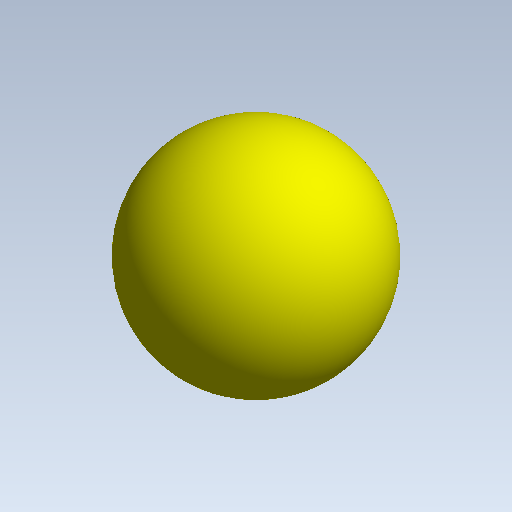
# Autodesk Inventor part: 17-40-27.4-12-ybrg1-43-6.747-28.5
Saved by Autodesk Inventor 2020 (Build 240168000, 168)
## iProperties
Part Number: 17-40-27.4-12-ybrg1-43-6.747-28.5
Material: Generic
Catalog Web Link: www.cadenas.de
Description: Ball for Y units-Y-bearings
Vendor: SKF
Document SubType Name: Modeling
Designer: partserver
Manufacturer: SKF
Mass: 0.160817 g
Surface Area: 1.43012 cm^2
Volume: 0.160817 cm^3
Density: 1 g/cm^3
Appearance: PSOLRGB-255-255-0
Category: PARTsolutions
Company: SKF
PSOL_IDENT_0: {$CADENAS_DATA\23d-libs\skf\bearings_units_and_housings\bearing_units\ball_bearing_units\y-unit_acce
PSOL_IDENT_1: ssories\ball.prj},218 {VTYP=3D},{NB=17-40-27.4-12-ybrg1-43-6.747-28.5},{LINA=17-40-27.4-12-ybrg1-43-
PSOL_IDENT_2: 6.747-28.5},{NN=Ball for Y units},{DATE=20.08.2020 13:45:09},{GEOMDATE=29.07.2020 16:06:32},{VERSION=
PSOL_IDENT_3: },{LINEID=1230},{WBVAR=},{WBNUMERIC=}  {NB=17-40-27.4-12-ybrg1-43-6.747-28.5},{LINA=17-40-27.4-12-yb
PSOL_IDENT_4: rg1-43-6.747-28.5},{KT=DUMMY},{DD=17.0000},{D=40},{B=27.400},{C=12.000},{PITCH=28.500},{DW=6.747},{F
PSOL_IDENT_5: O=IEC_BBY_006},{DESIGN=ybrg1},{X=0},{PN=43}
NB: 17-40-27.4-12-ybrg1-43-6.747-28.5
NN: Ball for Y units
NT: Y-bearings
NBSYN: $DD.-$D.-$B.-$C.-$DESIGN.-$PN.-$DW.-$PITCH.
LINA: 17-40-27.4-12-ybrg1-43-6.747-28.5
CATALOG: SKF
DD: 17
D: 40
B: 27.4
C: 12
PITCH: 28.5
DW: 6.747
FO: IEC_BBY_006
DESIGN: ybrg1
SUPPLIER: SKF
ARTICLENO: 17-40-27.4-12-ybrg1-43-6.747-28.5
BOMINFO: 17-40-27.4-12-ybrg1-43-6.747-28.5
CREATOR: CADENAS GmbH
Title: 17-40-27.4-12-ybrg1-43-6.747-28.5
Author: Cadenas PARTsolutions
Comments: Y-bearings
Autodesk Inventor part; units mm, degrees
sketch "Sketch_1" plane through (0, 0, 0) normal (0, 0, 1) x (1, 0, 0)
  line L0 (3.3735, 14.25) -> (-3.3735, 14.25)
  arc A0 (3.3735, 14.25) -> (-3.3735, 14.25) centre (0, 14.25) ccw
  line L1 (3.3735, 14.25) -> (-3.3735, 14.25)
  constraints: 4 end point, 2 point on circle, 1 centre point
revolve "Revolution1" add sketch "Sketch_1" angle 360 about axis through (3.3735, 14.25, 0) along (1, 0, 0)
ref_plane "ball_XY" through (0, 14.25, 0) normal (1, 0, 0) x (0, 0, -1)
ref_plane "ball_YZ" through (0, 14.25, 0) normal (0, 0, -1) x (0, 1, 0)
ref_plane "ball_ZX" through (0, 14.25, 0) normal (0, 1, 0) x (1, 0, 0)
body "Solid1"
